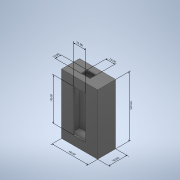
# Autodesk Inventor part: Корпус
Saved by Autodesk Inventor 2020 (Build 240168000, 168)
## iProperties
Created: 2023-05-10
Part Number: Корпус
Material: Полиацеталь, черный
Document SubType Name: Modeling
Designer: avoev
Density: 1.425 g/cm^3
Appearance: Гладкая — черная
Author: avoev
Autodesk Inventor part; units mm, degrees
ref_plane "YZ Plane" through (0, 0, 0) normal (1, 0, 0) x (0, 1, 0)
ref_plane "XZ Plane" through (0, 0, 0) normal (0, 1, 0) x (-1, 0, 0)
ref_plane "XY Plane" through (0, 0, 0) normal (0, 0, 1) x (1, 0, 0)
sketch "Эскиз1" plane through (0, 0, 0) normal (0, 0, 1) x (1, 0, 0)
  line L0 (0, 0) -> (60, 0)
  line L1 (60, 0) -> (60, -100)
  line L2 (60, -100) -> (0, -100)
  line L3 (0, -100) -> (0, 0)
  line L4 (2, -2) -> (58, -2)
  line L5 (58, -2) -> (58, -98)
  line L6 (58, -98) -> (2, -98)
  line L7 (2, -98) -> (2, -2)
  line L8 (0, 0) -> (60, -100) construction
  line L9 (60, 0) -> (0, -100) construction
  line L10 (2, -2) -> (58, -98) construction
  line L11 (58, -2) -> (2, -98) construction
  line L12 (20, -15) -> (40, -15)
  line L13 (40, -15) -> (40, -85)
  line L14 (40, -85) -> (20, -85)
  line L15 (20, -85) -> (20, -15)
  line L16 (20, -15) -> (40, -85) construction
  line L17 (40, -15) -> (20, -85) construction
  point P0 (30, -50)
  point P1 (30, -50)
  dimension "d0" = 60
  dimension "d1" = 100
  dimension "d2" = 56
  dimension "d3" = 96
  dimension "d8" = 20
  dimension "d9" = 70
  constraints: 36 end point, 6 parallel, 4 midpoint, 3 horizontal, 3 perpendicular
  measures "d0" distance of L1.end L2.end
  measures "d1" distance of L0.end L1.end
  measures "d2" distance of L5.end L6.end
  measures "d3" distance of L4.end L5.end
  measures "d8" distance of L13.end L14.end
  measures "d9" distance of L12.end L13.end
extrude "Выдавливание1" add sketch "Эскиз1" along normal blind 30 contours L0 L1 L2 L3 | L4 L5 L6 L7 | L12 L13 L14 L15
extrude "Выдавливание2" cut sketch "Эскиз1" along normal blind 28 contours L4 L5 L6 L7 | L12 L13 L14 L15
extrude "Выдавливание3" add sketch "Эскиз1" along normal blind 30 contours L12 L13 L14 L15
extrude "Выдавливание4" cut sketch "Эскиз1" along normal blind 35 contours L12 L13 L14 L15
sketch "Эскиз2" plane through (0, 0, 0) normal (0, 1, 0) x (-1, 0, 0)
  line L0 (-60, 0) -> (-60, 30) projected
  line L1 (-60, 30) -> (0, 30) projected
  line L2 (-60, 0) -> (0, 30) construction
  line L3 (-60, 0) -> (0, 0) projected
  line L4 (-60, 30) -> (0, 0) construction
  line L5 (-37.5, 20) -> (-22.5, 20)
  line L6 (-22.5, 20) -> (-22.5, 10)
  line L7 (-22.5, 10) -> (-37.5, 10)
  line L8 (-37.5, 10) -> (-37.5, 20)
  line L9 (-37.5, 20) -> (-22.5, 10) construction
  line L10 (-22.5, 20) -> (-37.5, 10) construction
  circle A0 centre (-30, 15) radius 2.5
  dimension "d14" = 15
  dimension "d15" = 10
  dimension "d16" = 5
  constraints: 16 end point, 2 midpoint, 2 parallel, 1 centre point, 1 coincident, 1 horizontal, 1 perpendicular
  measures "d14" distance of L6.end L7.end
  measures "d15" distance of L5.end L6.end
  measures "d16" diameter of A0
extrude "Выдавливание5" cut sketch "Эскиз2" along normal mid plane 100 contours L5 L6 L7 L8 | A0
extrude "Выдавливание6" cut sketch "Эскиз2" against normal through all contours A0
extrude "Выдавливание9" add sketch "Эскиз1" along normal blind 2 contours L0 L1 L2 L3 | L4 L5 L6 L7 | L12 L13 L14 L15
